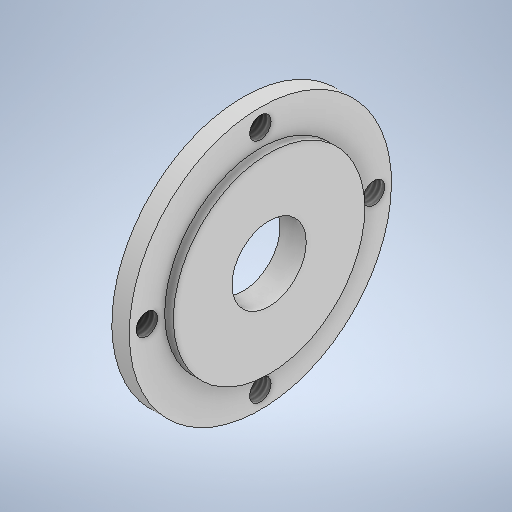
# Autodesk Inventor part: bielle côté 0
Saved by Autodesk Inventor 2025.2 (Build 292293000, 293)
## iProperties
Created: 2026-03-16
Part Number: bielle côté 0
Material: Générique
Document SubType Name: Modeling
Designer: genon
Density: 1 g/cm^3
Appearance: Par défaut
Author: genon
Autodesk Inventor part; units mm, degrees
ref_plane "YZ Plane" through (0, 0, 0) normal (1, 0, 0) x (0, 1, 0)
ref_plane "XZ Plane" through (0, 0, 0) normal (0, 1, 0) x (-1, 0, 0)
ref_plane "XY Plane" through (0, 0, 0) normal (0, 0, 1) x (1, 0, 0)
sketch "Esquisse1" plane through (0, 0, 0) normal (1, 0, 0) x (0, 1, 0)
  circle A0 centre (0, 0) radius 10.95
  circle A1 centre (0, 0) radius 15
  dimension "d0" = 21.9
  dimension "d1" = 30
  constraints: 2 centre point, 2 coincident
  measures "d0" diameter of A0
  measures "d1" diameter of A1
extrude "Extrusion1" add sketch "Esquisse1" along normal blind 2
sketch "Esquisse2" plane through (2, 0, 0) normal (1, 0, 0) x (0, 0, -1)
  circle A0 centre (0, 0) radius 10.95
  circle A1 centre (0, 0) radius 10.95
  constraints: 2 centre point, 2 coincident, 1 concentric
extrude "Extrusion2" add sketch "Esquisse2" along normal blind 1
sketch "Esquisse3" plane through (2, 0, 0) normal (1, 0, 0) x (0, 0, -1)
  line L0 (0, 0) -> (-13, 0)
  line L1 (0, 0) -> (0, 13)
  line L2 (0, 0) -> (13, 0) construction
  point P0 (0, -13)
  dimension "d6" = 13
  dimension "d7" = 13
  dimension "d8" = 90
  constraints: 6 end point, 2 coincident, 2 horizontal, 2 symmetric about line, 1 perpendicular, 1 vertical
  measures "d6" distance of L0.start L0.end
  measures "d7" distance of L0.start L1.end
  measures "d8" angle of L2 L1
hole "Perçage1" at (2, 13, 0) at (2, 0, 13) at (2, -13, 0) at (2, 0, -13) direction (-1, 0, 0) diameter 2.459 end through all thread size "M3x0.5" class "6H" standard "ISO Metric profile"
sketch "Esquisse4" plane through (2, 0, 0) normal (-1, 0, 0) x (0, 0, 1)
  circle A0 centre (0, 0) radius 10.95
  circle A1 centre (0, 0) radius 4.25
  dimension "d18" = 8.5
  constraints: 2 centre point, 2 coincident
  measures "d18" diameter of A1
extrude "Extrusion3" add sketch "Esquisse4" along normal up to surface (2 mm away)
sketch "Esquisse5" plane through (2, 0, 0) normal (-1, 0, 0) x (0, 0, 1)
  circle A0 centre (0, 0) radius 4.25
  dimension "d19" = 8.5
  constraints: 1 centre point, 1 coincident
  measures "d19" diameter of A0
extrude "Extrusion4" cut sketch "Esquisse5" against normal blind 10
